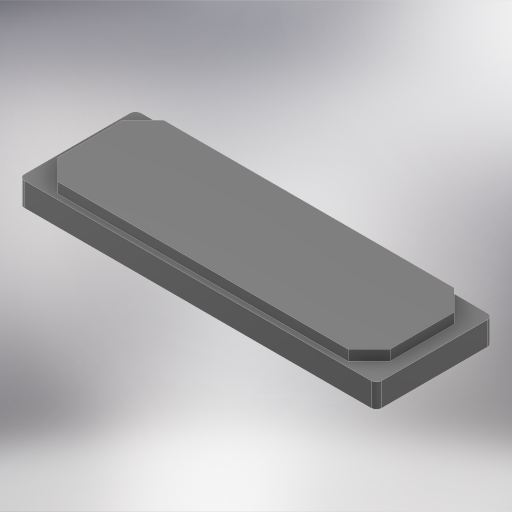
# Autodesk Inventor part: Speka
Saved by Autodesk Inventor 2024 (Build 280153000, 153)
## iProperties
Created: 2024-09-20
Part Number: Speka
Material: Acetal Resin, Black
Document SubType Name: Modeling
Designer: User
Density: 1.425 g/cm^3
Appearance: Smooth - Black
Author: User
Autodesk Inventor part; units mm, degrees
ref_plane "YZ Plane" through (0, 0, 0) normal (1, 0, 0) x (0, 1, 0)
ref_plane "XZ Plane" through (0, 0, 0) normal (0, 1, 0) x (-1, 0, 0)
ref_plane "XY Plane" through (0, 0, 0) normal (0, 0, 1) x (1, 0, 0)
sketch "Sketch1" plane through (0, 0, 0) normal (0, 1, 0) x (-1, 0, 0)
  line L0 (0, 0) -> (34, 0)
  line L1 (34, 0) -> (34, -11.1)
  line L2 (34, -11.1) -> (0, -11.1)
  line L3 (0, -11.1) -> (0, 0)
  dimension "d0" = 34
  dimension "d1" = 11.1
  constraints: 8 end point, 2 parallel, 1 horizontal, 1 perpendicular
  measures "d0" distance of L1.end L2.end
  measures "d1" distance of L0.end L1.end
extrude "Extrusion1" add sketch "Sketch1" along normal blind 3.5
sketch "Sketch2" plane through (0, 3.5, 0) normal (0, 1, 0) x (1, 0, 0)
  line L0 (-32.8, 0.5) -> (-1.2, 0.5)
  line L1 (-1.2, 0.5) -> (-1.2, 10.6)
  line L2 (-1.2, 10.6) -> (-32.8, 10.6)
  line L3 (-32.8, 10.6) -> (-32.8, 0.5)
  line L4 (-34, 11.1) -> (-34, 0) projected
  line L5 (0, 0) -> (0, 11.1) projected
  line L6 (0, 11.1) -> (-34, 11.1) projected
  line L7 (-34, 0) -> (0, 0) projected
  dimension "d4" = 1.2
  dimension "d5" = 1.2
  dimension "d6" = 0.5
  dimension "d7" = 0.5
  constraints: 8 end point, 2 parallel, 1 horizontal, 1 perpendicular
  measures "d4" distance between parallel lines of L4 L3
  measures "d5" distance between parallel lines of L5 L1
  measures "d6" distance between parallel lines of L6 L2
  measures "d7" distance between parallel lines of L7 L0
extrude "Extrusion2" cut sketch "Sketch2" against normal blind 1
sketch "Sketch3" plane through (0, 0, 0) normal (0, -1, 0) x (1, 0, 0)
  line L0 (-0.55, -10.5) -> (-33.45, -10.5)
  line L1 (-33.45, -10.5) -> (-33.45, -0.6)
  line L2 (-33.45, -0.6) -> (-0.55, -0.6)
  line L3 (-0.55, -0.6) -> (-0.55, -10.5)
  line L4 (-0.55, -10.5) -> (-33.45, -0.6) construction
  line L5 (-33.45, -10.5) -> (-0.55, -0.6) construction
  line L6 (-17, -5.55) -> (-17, -7.3465)
  line L7 (-17, -7.3465) -> (-17, -5.55)
  line L8 (-22.3316, -5.55) -> (-22.3865, -5.55)
  line L9 (-22.3865, -5.55) -> (-17, -5.55)
  line L10 (-34, -11.1) -> (-34, 0) projected
  line L11 (0, -11.1) -> (-34, -11.1) projected
  line L12 (0, -11.1) -> (-34, -11.1) projected
  line L13 (0, 0) -> (0, -11.1) projected
  line L14 (-34, 0) -> (0, 0) projected
  line L15 (-34, -11.1) -> (-34, 0) projected
  point P0 (-34, -5.55)
  point P1 (-17, -11.1)
  dimension "d10" = 32.9
  dimension "d11" = 9.9
  constraints: 20 end point, 4 midpoint, 2 collinear, 2 horizontal, 2 parallel, 2 point on line, 1 perpendicular, 1 vertical
  measures "d10" distance of L1.end L2.end
  measures "d11" distance of L0.end L1.end
extrude "Extrusion3" cut sketch "Sketch3" against normal blind 0.25
fillet "Fillet1" radius 2 4 edges at (-33.45, 0.125, -10.5) (-33.45, 0.125, -0.6) (-0.55, 0.125, -0.6) (-0.55, 0.125, -10.5)
fillet "Fillet2" radius 0.5 4 edges at (-34, 1.375, 0) (-34, 1.375, -11.1) (0, 1.375, 0) (0, 1.375, -11.1)
chamfer "Chamfer1" distance 2 angle 45 4 edges at (-1.2, 3, -0.5) (-1.2, 3, -10.6) (-32.8, 3, -0.5) (-32.8, 3, -10.6)
equation "\"d5\" = d4"
equation "\"d7\" = d6"
body "Solid1"
